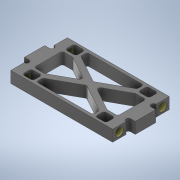
# Autodesk Inventor part: Head_diagonal
Saved by Autodesk Inventor 2020 (Build 240168000, 168)
## iProperties
Part Number: Head_diagonal
Material: アセタール樹脂、黒
Document SubType Name: Modeling
Designer: Masato Kubotera
Density: 1.425 g/cm^3
Appearance: 滑らか - 黒
Description: POM T5
Mass: 3.41927 g
Surface Area: 32.3587 cm^2
Volume: 2.39949 cm^3
Author: Masato Kubotera
Autodesk Inventor part; units mm, degrees
ref_plane "YZ Plane" through (0, 0, 0) normal (1, 0, 0) x (0, 1, 0)
ref_plane "XZ Plane" through (0, 0, 0) normal (0, 1, 0) x (-1, 0, 0)
ref_plane "XY Plane" through (0, 0, 0) normal (0, 0, 1) x (1, 0, 0)
sketch "スケッチ1" plane through (0, 0, 0) normal (0, 0, 1) x (1, 0, 0)
  line L0 (-12.5, -22.5) -> (-12.5, 22.5)
  line L1 (-12.5, 22.5) -> (12.5, 22.5)
  line L2 (12.5, 22.5) -> (12.5, -22.5)
  line L3 (12.5, -22.5) -> (-12.5, -22.5)
  line L4 (-12.5, -22.5) -> (12.5, 22.5) construction
  line L5 (-12.5, 22.5) -> (12.5, -22.5) construction
  line L6 (0, -22.5) -> (0, 22.5) construction
  line L7 (-12.5, 0) -> (12.5, 0) construction
  line L8 (-4.5, -22.5) -> (-4.5, -24.5)
  line L9 (-4.5, -24.5) -> (4.5, -24.5)
  arc A0 (-4.5, -22.5) -> (-6.6, -22.5) centre (-5.55, -22.5) ccw
  line L10 (-9.5, -22.5) -> (-9.5, -18.5) construction
  line L11 (-11.5, -22.5) -> (-11.5, -18.5) construction
  line L12 (-11.5, -18.5) -> (-7.5, -18.5) construction
  line L13 (-7.5, -18.5) -> (-7.5, -22.5) construction
  line L14 (4.5, -22.5) -> (4.5, -24.5)
  arc A1 (6.6, -22.5) -> (4.5, -22.5) centre (5.55, -22.5) ccw
  line L15 (9.5, -22.5) -> (9.5, -18.5) construction
  line L16 (11.5, -22.5) -> (11.5, -18.5) construction
  line L17 (11.5, -18.5) -> (7.5, -18.5) construction
  line L18 (7.5, -18.5) -> (7.5, -22.5) construction
  line L19 (-8.5, -13.75) -> (-10.5, -13.75)
  line L20 (-11.5, -14.75) -> (-11.5, -17.5)
  line L21 (-10.5, -18.5) -> (-8.5, -18.5)
  line L22 (-7.5, -17.5) -> (-7.5, -14.75)
  line L23 (-7.5, -13.75) -> (-11.5, -18.5) construction
  line L24 (-11.5, -13.75) -> (-7.5, -18.5) construction
  arc A2 (-11.5, -17.5) -> (-10.5, -18.5) centre (-10.5, -17.5) ccw
  arc A3 (-8.5, -18.5) -> (-7.5, -17.5) centre (-8.5, -17.5) ccw
  arc A4 (-7.5, -14.75) -> (-8.5, -13.75) centre (-8.5, -14.75) ccw
  arc A5 (-10.5, -13.75) -> (-11.5, -14.75) centre (-10.5, -14.75) ccw
  line L25 (-6.25, -17.5) -> (-6.25, -14.083)
  line L26 (-6.1242, -13.5974) -> (-0.8742, -4.1474)
  line L27 (-5.25, -18.5) -> (0, -18.5)
  arc A6 (-6.1242, -13.5974) -> (-6.25, -14.083) centre (-5.25, -14.083) ccw
  arc A7 (-6.25, -17.5) -> (-5.25, -18.5) centre (-5.25, -17.5) ccw
  line L28 (-12.5, 0) -> (12.5, 0)
  line L29 (6.25, -17.5) -> (6.25, -14.083)
  line L30 (6.1242, -13.5974) -> (0.8742, -4.1474)
  line L31 (5.25, -18.5) -> (0, -18.5)
  arc A8 (6.25, -14.083) -> (6.1242, -13.5974) centre (5.25, -14.083) ccw
  arc A9 (5.25, -18.5) -> (6.25, -17.5) centre (5.25, -17.5) ccw
  arc A10 (0.8742, -4.1474) -> (-0.8742, -4.1474) centre (0, -4.633) ccw
  line L32 (8.5, -13.75) -> (10.5, -13.75)
  line L33 (11.5, -14.75) -> (11.5, -17.5)
  line L34 (10.5, -18.5) -> (8.5, -18.5)
  line L35 (7.5, -17.5) -> (7.5, -14.75)
  arc A11 (10.5, -18.5) -> (11.5, -17.5) centre (10.5, -17.5) ccw
  arc A12 (8.5, -13.75) -> (7.5, -14.75) centre (8.5, -14.75) ccw
  arc A13 (11.5, -14.75) -> (10.5, -13.75) centre (10.5, -14.75) ccw
  arc A14 (7.5, -17.5) -> (8.5, -18.5) centre (8.5, -17.5) ccw
  line L36 (1.6998, -0.4856) -> (8.0886, -11.9856)
  line L37 (8.9628, -12.5) -> (10.25, -12.5)
  line L38 (11.25, -11.5) -> (11.25, 0)
  line L39 (1.6998, 0.4856) -> (8.0886, 11.9856)
  line L40 (8.9628, 12.5) -> (10.25, 12.5)
  line L41 (11.25, 11.5) -> (11.25, 0)
  arc A15 (1.6998, 0.4856) -> (1.6998, -0.4856) centre (2.5739, 0) ccw
  arc A16 (8.0886, -11.9856) -> (8.9628, -12.5) centre (8.9628, -11.5) ccw
  arc A17 (10.25, -12.5) -> (11.25, -11.5) centre (10.25, -11.5) ccw
  arc A18 (11.25, 11.5) -> (10.25, 12.5) centre (10.25, 11.5) ccw
  arc A19 (8.9628, 12.5) -> (8.0886, 11.9856) centre (8.9628, 11.5) ccw
  line L42 (-1.6998, -0.4856) -> (-8.0886, -11.9856)
  line L43 (-8.9628, -12.5) -> (-10.25, -12.5)
  line L44 (-11.25, -11.5) -> (-11.25, 0)
  line L45 (-11.25, 11.5) -> (-11.25, 0)
  line L46 (-8.9628, 12.5) -> (-10.25, 12.5)
  line L47 (-1.6998, 0.4856) -> (-8.0886, 11.9856)
  arc A20 (-1.6998, -0.4856) -> (-1.6998, 0.4856) centre (-2.5739, 0) ccw
  arc A21 (-8.9628, -12.5) -> (-8.0886, -11.9856) centre (-8.9628, -11.5) ccw
  arc A22 (-11.25, -11.5) -> (-10.25, -12.5) centre (-10.25, -11.5) ccw
  arc A23 (-10.25, 12.5) -> (-11.25, 11.5) centre (-10.25, 11.5) ccw
  arc A24 (-8.0886, 11.9856) -> (-8.9628, 12.5) centre (-8.9628, 11.5) ccw
  point P0 (0, 0)
  point P1 (4.5, -22.5)
  point P2 (6.6, -22.5)
  point P3 (4.5, -22.5)
  point P4 (-9.5, -16.125)
  point P5 (-9.5, -16.125)
  point P6 (0, -2.5739)
  point P7 (1.4299, 0)
  point P8 (8.3744, -12.5)
  point P9 (11.25, -12.5)
  point P10 (8.3744, 12.5)
  point P11 (11.25, 12.5)
  point P12 (1.5739, 0)
  point P13 (-1.5739, 0)
  point P14 (-11.25, 0)
  dimension "d0" = 4
  dimension "d1" = 4
  dimension "d2" = 1.05
  dimension "d3" = 19
  dimension "d4" = 9
  dimension "d5" = 25
  dimension "d7" = 2
  dimension "d8" = 45
  dimension "d35" = 1
  dimension "d36" = 4
  dimension "d38" = 1.25
  dimension "d42" = 1
  dimension "d44" = 1
  dimension "d47" = 1.25
  dimension "d48" = 2.5
  dimension "d49" = 1.25
  dimension "d50" = 1
  dimension "d51" = 4.75
  constraints: 94 end point, 50 point on circle, 46 symmetric about line, 25 centre point, 25 point on line, 24 tangent, 9 midpoint, 8 equal radius, 6 perpendicular, 5 parallel, 4 vertical, 2 collinear, 2 horizontal, 23 other
  measures "d0" distance of L10.end L10.start
  measures "d1" distance of L11.end L12.end
  measures "d2" radius of A0
  measures "d3" distance of L15.start L10.start
  measures "d4" distance of L8.end L9.end
  measures "d5" distance of L2.end L0.start
  measures "d7" distance of L8.start L8.end
  measures "d8" distance of L0.start L0.end
  measures "d35" radius of A2
  measures "d36" distance between parallel lines of L22 L20
  measures "d38" distance between parallel lines of L25 L22
  measures "d42" radius of A6
  measures "d44" radius of A10
  measures "d47" distance between parallel lines of L32 L37
  measures "d48" distance between parallel lines of L30 L36
  measures "d49" distance between parallel lines of L2 L38
  measures "d50" radius of A15
  measures "d51" distance between parallel lines of L21 L19
extrude "押し出し1" add sketch "スケッチ1" along normal blind 5 contours L0 L28 L44 A22 L43 A21 L42 A20 A15 L36 A16 L37 A17 L38 L2 L3 A1 A0 | L3 L14 L9 L8
sketch "スケッチ2" plane through (-12.5, -22.5, 0) normal (0, -1, 0) x (1, 0, 0)
  line L0 (12.5, 5) -> (12.5, 0)
  line L1 (0, 0) -> (5.9, 0) projected
  line L2 (8, 5) -> (5.9, 5) projected
  point P0 (3, 2.5)
  point P1 (22, 2.5)
  point P2 (17, 5)
  dimension "d22" = 2.5
  dimension "d30" = 19
  constraints: 2 end point, 1 point on line, 1 symmetric about line, 1 vertical
  measures "d22" distance from line of L1 point (3, 2.5)
  measures "d30" distance of point (22, 2.5) point (3, 2.5)
hole "穴1" at (-9.5, -22.5, 2.5) at (9.5, -22.5, 2.5) direction (0, 1, 0) diameter 3.4587 depth 5 tip angle 118 thread size "M4x0.5" class "6H" standard "ISO Metric profile"
mirror "ミラー1" about plane through (12.5, 0, 0) normal (0, 1, 0)
equation "\"d38\" = d11"
equation "\"d30\" = d3"
equation "\"d11\" = 1.25"
